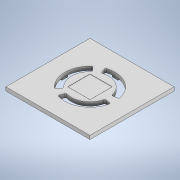
# Autodesk Inventor part: CubeFace
Saved by Autodesk Inventor 2022 (Build 260153000, 153)
## iProperties
Created: 2022-04-08
Part Number: CubeFace
Material: Generic
Document SubType Name: Modeling
Designer: awp
Density: 1 g/cm^3
Appearance: Default
Author: awp
Autodesk Inventor part; units mm, degrees
ref_plane "YZ Plane" through (0, 0, 0) normal (1, 0, 0) x (0, 1, 0)
ref_plane "XZ Plane" through (0, 0, 0) normal (0, 1, 0) x (-1, 0, 0)
ref_plane "XY Plane" through (0, 0, 0) normal (0, 0, 1) x (1, 0, 0)
sketch "Sketch1" plane through (0, 0, 0) normal (0, 1, 0) x (-1, 0, 0)
  line L0 (0, 0) -> (57.5, 0)
  line L1 (57.5, 0) -> (57.5, -57.5)
  line L2 (57.5, -57.5) -> (0, -57.5)
  line L3 (0, -57.5) -> (0, 0)
  dimension "d0" = 57.5
  dimension "d1" = 57.5
  constraints: 8 end point, 2 parallel, 1 horizontal, 1 perpendicular
  measures "d0" distance of L1.end L2.end
  measures "d1" distance of L0.end L1.end
extrude "Extrusion1" add sketch "Sketch1" along normal blind 2.54
sketch "Sketch2" plane through (0, 0, 0) normal (0, -1, 0) x (1, 0, 0)
  line L0 (0, -57.5) -> (-57.5, -57.5) projected
  line L1 (0, 0) -> (0, -57.5) projected
  line L2 (-57.5, 0) -> (0, 0) projected
  line L3 (-57.5, -57.5) -> (-57.5, 0) projected
  line L4 (-57.5, -57.5) -> (-57.5, 0) projected
  line L5 (-57.5, -57.5) -> (-38.3333, -57.5)
  line L6 (-38.3333, -57.5) -> (-38.3333, -38.3333)
  line L7 (-38.3333, -38.3333) -> (-57.5, -38.3333)
  line L8 (-57.5, -38.3333) -> (-57.5, -57.5)
  line L9 (-57.5, -38.3333) -> (-38.3333, -38.3333)
  line L10 (-38.3333, -38.3333) -> (-38.3333, -19.1667)
  line L11 (-38.3333, -19.1667) -> (-57.5, -19.1667)
  line L12 (-57.5, -19.1667) -> (-57.5, -38.3333)
  line L13 (-57.5, 0) -> (0, 0) projected
  line L14 (-57.5, -19.1667) -> (-38.3333, -19.1667)
  line L15 (-38.3333, -19.1667) -> (-38.3333, 0)
  line L16 (-38.3333, 0) -> (-57.5, 0)
  line L17 (-57.5, 0) -> (-57.5, -19.1667)
  line L18 (-38.3333, 0) -> (-19.1667, 0)
  line L19 (-19.1667, 0) -> (-19.1667, -19.1667)
  line L20 (-19.1667, -19.1667) -> (-38.3333, -19.1667)
  line L21 (-38.3333, -19.1667) -> (-38.3333, 0)
  line L22 (-19.1667, -19.1667) -> (0, -19.1667)
  line L23 (0, -19.1667) -> (0, 0)
  line L24 (0, 0) -> (-19.1667, 0)
  line L25 (-19.1667, 0) -> (-19.1667, -19.1667)
  line L26 (-19.1667, -19.1667) -> (-38.3333, -19.1667)
  line L27 (-38.3333, -19.1667) -> (-38.3333, -38.3333)
  line L28 (-38.3333, -38.3333) -> (-19.1667, -38.3333)
  line L29 (-19.1667, -38.3333) -> (-19.1667, -19.1667)
  line L30 (-19.1667, -38.3333) -> (-38.3333, -38.3333)
  line L31 (-38.3333, -38.3333) -> (-38.3333, -57.5)
  line L32 (-38.3333, -57.5) -> (-19.1667, -57.5)
  line L33 (-19.1667, -57.5) -> (-19.1667, -38.3333)
  line L34 (0, -19.1667) -> (-19.1667, -19.1667)
  line L35 (-19.1667, -19.1667) -> (-19.1667, -38.3333)
  line L36 (-19.1667, -38.3333) -> (0, -38.3333)
  line L37 (0, -38.3333) -> (0, -19.1667)
  line L38 (0, -38.3333) -> (-19.1667, -38.3333)
  line L39 (-19.1667, -38.3333) -> (-19.1667, -57.5)
  line L40 (-19.1667, -57.5) -> (0, -57.5)
  line L41 (0, -57.5) -> (0, -38.3333)
  line L42 (0, -57.5) -> (-57.5, -57.5) projected
  line L43 (-57.5, -57.5) -> (-49.88, -57.5)
  line L44 (-49.88, -57.5) -> (-49.88, -49.88)
  line L45 (-49.88, -49.88) -> (-57.5, -49.88)
  line L46 (-57.5, -49.88) -> (-57.5, -57.5)
  line L47 (-38.3333, -38.3333) -> (-45.9533, -38.3333)
  line L48 (-45.9533, -38.3333) -> (-45.9533, -45.9533)
  line L49 (-45.9533, -45.9533) -> (-38.3333, -45.9533)
  line L50 (-38.3333, -45.9533) -> (-38.3333, -38.3333)
  line L51 (-45.9533, -45.9533) -> (-49.88, -45.9533)
  line L52 (-49.88, -45.9533) -> (-49.88, -49.88)
  line L53 (-49.88, -49.88) -> (-45.9533, -49.88)
  line L54 (-45.9533, -49.88) -> (-45.9533, -45.9533)
  line L55 (-49.88, -26.7867) -> (-49.88, -30.7133)
  line L56 (-49.88, -30.7133) -> (-45.9533, -30.7133)
  line L57 (-45.9533, -26.7867) -> (-49.88, -26.7867)
  line L58 (-45.9533, -30.7133) -> (-45.9533, -26.7867)
  line L59 (-49.88, -7.62) -> (-49.88, -11.5467)
  line L60 (-49.88, -11.5467) -> (-45.9533, -11.5467)
  line L61 (-45.9533, -7.62) -> (-49.88, -7.62)
  line L62 (-45.9533, -11.5467) -> (-45.9533, -7.62)
  line L63 (-30.7133, -45.9533) -> (-30.7133, -49.88)
  line L64 (-30.7133, -49.88) -> (-26.7867, -49.88)
  line L65 (-26.7867, -45.9533) -> (-30.7133, -45.9533)
  line L66 (-26.7867, -49.88) -> (-26.7867, -45.9533)
  line L67 (-30.7133, -26.7867) -> (-30.7133, -30.7133)
  line L68 (-30.7133, -30.7133) -> (-26.7867, -30.7133)
  line L69 (-26.7867, -26.7867) -> (-30.7133, -26.7867)
  line L70 (-26.7867, -30.7133) -> (-26.7867, -26.7867)
  line L71 (-30.7133, -7.62) -> (-30.7133, -11.5467)
  line L72 (-30.7133, -11.5467) -> (-26.7867, -11.5467)
  line L73 (-26.7867, -7.62) -> (-30.7133, -7.62)
  line L74 (-26.7867, -11.5467) -> (-26.7867, -7.62)
  line L75 (-11.5467, -45.9533) -> (-11.5467, -49.88)
  line L76 (-11.5467, -49.88) -> (-7.62, -49.88)
  line L77 (-7.62, -45.9533) -> (-11.5467, -45.9533)
  line L78 (-7.62, -49.88) -> (-7.62, -45.9533)
  line L79 (-11.5467, -26.7867) -> (-11.5467, -30.7133)
  line L80 (-11.5467, -30.7133) -> (-7.62, -30.7133)
  line L81 (-7.62, -26.7867) -> (-11.5467, -26.7867)
  line L82 (-7.62, -30.7133) -> (-7.62, -26.7867)
  line L83 (-11.5467, -7.62) -> (-11.5467, -11.5467)
  line L84 (-11.5467, -11.5467) -> (-7.62, -11.5467)
  line L85 (-7.62, -7.62) -> (-11.5467, -7.62)
  line L86 (-7.62, -11.5467) -> (-7.62, -7.62)
  dimension "d4" = 19.1667
  dimension "d5" = 19.1667
  dimension "d6" = 19.1667
  dimension "d7" = 19.1667
  dimension "d8" = 19.1667
  dimension "d9" = 7.62
  dimension "d10" = 7.62
  dimension "d11" = 7.62
  dimension "d12" = 7.62
  dimension "d15" = 19.1667
  dimension "d18" = 19.1667
  constraints: 160 end point, 24 parallel, 13 horizontal, 12 perpendicular, 2 collinear, 2 point on line, 1 vertical, 62 other
  measures "d4" distance of L7.end L6.end
  measures "d5" distance of L5.end L6.end
  measures "d6" distance of L10.end L11.end
  measures "d7" distance of L9.end L10.end
  measures "d8" distance of L19.end L20.end
  measures "d9" distance of L45.end L44.end
  measures "d10" distance of L44.end L43.end
  measures "d11" distance of L49.end L48.end
  measures "d12" distance of L48.end L47.end
  measures "d15" distance of L51.end L55.start
  measures "d18" distance of L51.end L63.start
extrude "Extrusion2" add sketch "Sketch2" along normal blind 1.27 contours L52 L51 L54 L53 | L57 L58 L56 L55 | L61 L62 L60 L59 | L65 L66 L64 L63 | L69 L70 L68 L67 | L73 L74 L72 L71 | L77 L78 L76 L75 | L81 L82 L80 L79 | L85 L86 L84 L83
chamfer "Chamfer1" [suppressed]
sketch "Sketch3" plane through (0, 2.54, 0) normal (0, 1, 0) x (1, 0, 0)
  line L0 (0, 57.5) -> (-57.5, 57.5) projected
  line L1 (-57.5, 57.5) -> (-57.5, 0) projected
  line L2 (-57.5, 0) -> (0, 0) projected
  line L3 (0, 0) -> (0, 57.5) projected
  line L4 (-28.75, 28.75) -> (-36.37, 28.75)
  line L5 (-36.37, 28.75) -> (-36.37, 21.13)
  line L6 (-36.37, 21.13) -> (-28.75, 21.13)
  line L7 (-28.75, 21.13) -> (-28.75, 28.75)
  line L8 (-36.37, 21.13) -> (-21.13, 21.13)
  line L9 (-21.13, 21.13) -> (-21.13, 36.37)
  line L10 (-21.13, 36.37) -> (-36.37, 36.37)
  line L11 (-36.37, 36.37) -> (-36.37, 21.13)
  dimension "d26" = 7.62
  dimension "d27" = 7.62
  dimension "d30" = 15.24
  dimension "d31" = 15.24
  constraints: 16 end point, 4 parallel, 2 horizontal, 2 perpendicular
  measures "d26" distance of L6.end L5.end
  measures "d27" distance of L5.end L4.end
  measures "d30" distance of L10.end L9.end
  measures "d31" distance of L9.end L8.end
extrude "Extrusion3" cut sketch "Sketch3" against normal blind 0.127 contours L7 L6 L5 L4 | L4 L11 L10 L9 L8 L7
sketch "Sketch4" plane through (0, 0, 0) normal (0, -1, 0) x (1, 0, 0)
  line L0 (-49.88, -11.5467) -> (-49.88, -7.62) projected
  line L1 (-49.88, -7.62) -> (-45.9533, -7.62) projected
  line L2 (-45.9533, -7.62) -> (-45.9533, -11.5467) projected
  line L3 (-30.7133, -49.88) -> (-30.7133, -45.9533) projected
  line L4 (-30.7133, -45.9533) -> (-26.7867, -45.9533) projected
  line L5 (-26.7867, -45.9533) -> (-26.7867, -49.88) projected
  line L6 (-26.7867, -49.88) -> (-30.7133, -49.88) projected
  line L7 (-11.5467, -11.5467) -> (-11.5467, -7.62) projected
  line L8 (-11.5467, -7.62) -> (-7.62, -7.62) projected
  line L9 (-7.62, -7.62) -> (-7.62, -11.5467) projected
  line L10 (-7.62, -11.5467) -> (-11.5467, -11.5467) projected
  line L11 (-11.5467, -30.7133) -> (-11.5467, -26.7867) projected
  line L12 (-11.5467, -26.7867) -> (-7.62, -26.7867) projected
  line L13 (-7.62, -26.7867) -> (-7.62, -30.7133) projected
  line L14 (-7.62, -30.7133) -> (-11.5467, -30.7133) projected
  line L15 (-30.7133, -30.7133) -> (-30.7133, -26.7867) projected
  line L16 (-30.7133, -26.7867) -> (-26.7867, -26.7867) projected
  line L17 (-26.7867, -26.7867) -> (-26.7867, -30.7133) projected
  line L18 (-26.7867, -30.7133) -> (-30.7133, -30.7133) projected
  line L19 (-49.88, -30.7133) -> (-49.88, -26.7867) projected
  line L20 (-49.88, -26.7867) -> (-45.9533, -26.7867) projected
  line L21 (-45.9533, -26.7867) -> (-45.9533, -30.7133) projected
  line L22 (-45.9533, -30.7133) -> (-49.88, -30.7133) projected
  line L23 (-11.5467, -49.88) -> (-11.5467, -45.9533) projected
  line L24 (-11.5467, -45.9533) -> (-7.62, -45.9533) projected
  line L25 (-7.62, -45.9533) -> (-7.62, -49.88) projected
  line L26 (-7.62, -49.88) -> (-11.5467, -49.88) projected
  line L27 (-30.7133, -11.5467) -> (-30.7133, -7.62) projected
  line L28 (-30.7133, -7.62) -> (-26.7867, -7.62) projected
  line L29 (-26.7867, -7.62) -> (-26.7867, -11.5467) projected
  line L30 (-26.7867, -11.5467) -> (-30.7133, -11.5467) projected
  line L31 (-49.88, -45.9533) -> (-45.9533, -45.9533) projected
  line L32 (-45.9533, -45.9533) -> (-45.9533, -49.88) projected
  line L33 (-45.9533, -49.88) -> (-49.88, -49.88) projected
  line L34 (-49.88, -49.88) -> (-49.88, -45.9533) projected
  line L35 (0, -57.5) -> (-57.5, -57.5) projected
  line L36 (0, 0) -> (0, -57.5) projected
  line L37 (-57.5, 0) -> (0, 0) projected
  line L38 (-57.5, -57.5) -> (-57.5, 0) projected
  circle A0 centre (-28.75, -28.75) radius 17.2033
  circle A1 centre (-28.75, -28.75) radius 12.7
  line L39 (-28.75, -28.75) -> (-37.3517, -43.6485)
  line L40 (-28.75, -28.75) -> (-11.5467, -28.75) construction
  line L41 (-28.75, -28.75) -> (-37.3517, -13.8515)
  line L42 (-28.75, -28.75) -> (-11.5467, -28.75) construction
  line L43 (-28.75, -28.75) -> (-11.5467, -28.75)
  line L44 (-28.75, -28.75) -> (-11.5467, -28.75) construction
  line L45 (-28.75, -28.75) -> (-34.6339, -44.9158)
  line L46 (-28.75, -28.75) -> (-11.5467, -28.75) construction
  line L47 (-28.75, -28.75) -> (-39.8081, -41.9285)
  line L48 (-28.75, -28.75) -> (-11.5467, -28.75) construction
  line L49 (-28.75, -28.75) -> (-34.6339, -12.5842)
  line L50 (-28.75, -28.75) -> (-11.5467, -28.75) construction
  line L51 (-28.75, -28.75) -> (-39.8081, -15.5715)
  line L52 (-28.75, -28.75) -> (-11.5467, -28.75) construction
  line L53 (-28.75, -28.75) -> (-11.808, -31.7373)
  line L54 (-28.75, -28.75) -> (-11.5467, -28.75) construction
  line L55 (-28.75, -28.75) -> (-11.808, -25.7627)
  line L56 (-28.75, -28.75) -> (-11.5467, -28.75) construction
  line L57 (-45.9533, -11.5467) -> (-49.88, -11.5467) projected
  point P0 (-36.9134, -19.0212)
  point P1 (-36.9134, -38.4788)
  point P2 (-16.2429, -26.5447)
  point P3 (-33.0937, -16.8159)
  point P4 (-16.2429, -30.9553)
  point P5 (-33.0937, -40.6841)
  dimension "d32" = 25.4
  dimension "d35" = 120
  dimension "d36" = 120
  dimension "d37" = 0
  dimension "d38" = 110
  dimension "d39" = 130
  dimension "d40" = 110
  dimension "d41" = 130
  dimension "d42" = 10
  dimension "d43" = 10
  constraints: 36 end point, 10 horizontal, 9 equal length, 1 centre point, 1 coincident, 1 collinear, 10 other
  measures "d32" diameter of A1
  measures "d35" angle of L39 L40
  measures "d36" angle of L42 L41
  measures "d37" distance between parallel lines of L43 L44
  measures "d38" angle of L45 L46
  measures "d39" angle of L47 L48
  measures "d40" angle of L50 L49
  measures "d41" angle of L52 L51
  measures "d42" angle of L53 L54
  measures "d43" angle of L56 L55
extrude "Extrusion4" cut sketch "Sketch4" against normal through all contours A0 L45 A1 L53 | A0 L51 A1 L47 | L55 A1 L49 A0
fillet "Fillet1" radius 0.889 12 edges at (-11.808, 1.27, -25.7627) (-16.2429, 1.27, -26.5447) (-33.0937, 1.27, -16.8159) (-34.6339, 1.27, -12.5842) (-11.808, 1.27, -31.7373) (-16.2429, 1.27, -30.9553) (-34.6339, 1.27, -44.9158) (-33.0937, 1.27, -40.6841) (-36.9134, 1.27, -38.4788) (-39.8081, 1.27, -41.9285) (-36.9134, 1.27, -19.0212) (-39.8081, 1.27, -15.5715)
equation "\"d5\" = d4"
equation "\"d6\" = d4"
equation "\"d7\" = d4"
equation "\"d8\" = d4"
body "Solid1"
